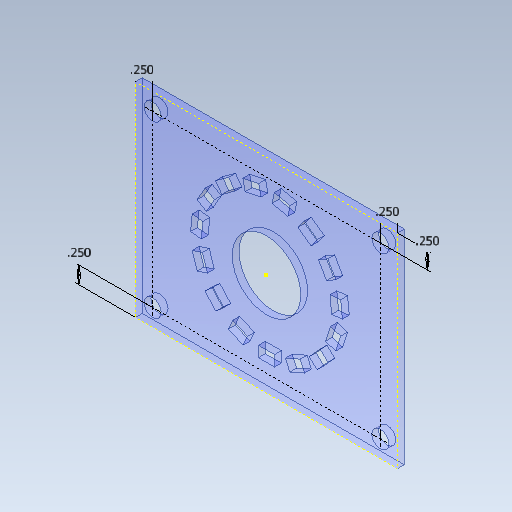
# Autodesk Inventor part: 2020LightRingCover
Saved by Autodesk Inventor 2020.2 (Build 242310000, 310)
## iProperties
Created: 2018-12-24
Part Number: 2020LightRingCover
Material: Polycarbonate, Clear
Document SubType Name: Modeling
Designer: steele
Density: 1.2 g/cm^3
Appearance: Clear - Blue
Author: steele
Comments: 1/11/19 Reduced the diamter of the outside by 2 mm so the part would fit better onto the main housing.
Autodesk Inventor part; units mm, degrees
ref_plane "YZ Plane" through (0, 0, 0) normal (1, 0, 0) x (0, 1, 0)
ref_plane "XZ Plane" through (0, 0, 0) normal (0, 1, 0) x (-1, 0, 0)
ref_plane "XY Plane" through (0, 0, 0) normal (0, 0, 1) x (1, 0, 0)
sketch "Sketch1" plane through (0, 0, 0) normal (0, 0, 1) x (1, 0, 0)
  circle A0 centre (0, 0) radius 34
  dimension "d0" = 68
  constraints: 1 centre point, 1 coincident
  measures "d0" diameter of A0
extrude "Extrusion1" add sketch "Sketch1" against normal blind 2.54
sketch "Sketch3" plane through (0, 0, -2.54) normal (0, 0, -1) x (-1, 0, 0)
  circle A0 centre (0, 0) radius 26 construction
  line L0 (3, -24) -> (-3, -24)
  line L1 (-3, -24) -> (-3, -28)
  line L2 (-3, -28) -> (3, -28)
  line L3 (3, -28) -> (3, -24)
  line L4 (3, -24) -> (-3, -28) construction
  line L5 (-3, -24) -> (3, -28) construction
  line L6 (8.648, -26.7995) -> (14.1293, -24.3591)
  line L7 (14.1293, -24.3591) -> (12.5023, -20.7049)
  line L8 (7.021, -23.1453) -> (8.648, -26.7995)
  line L9 (12.5023, -20.7049) -> (7.021, -23.1453)
  line L10 (18.8007, -20.9651) -> (22.8154, -16.5062)
  line L11 (22.8154, -16.5062) -> (19.8429, -13.8297)
  line L12 (15.8281, -18.2886) -> (18.8007, -20.9651)
  line L13 (19.8429, -13.8297) -> (15.8281, -18.2886)
  line L14 (25.7025, -11.5056) -> (27.5566, -5.7993)
  line L15 (27.5566, -5.7993) -> (23.7524, -4.5632)
  line L16 (21.8983, -10.2696) -> (25.7025, -11.5056)
  line L17 (23.7524, -4.5632) -> (21.8983, -10.2696)
  line L18 (28.1602, -0.0568) -> (27.533, 5.9104)
  line L19 (27.533, 5.9104) -> (23.5549, 5.4922)
  line L20 (24.1821, -0.4749) -> (28.1602, -0.0568)
  line L21 (23.5549, 5.4922) -> (24.1821, -0.4749)
  line L22 (25.7487, 11.4019) -> (22.7487, 16.5981)
  line L23 (22.7487, 16.5981) -> (19.2846, 14.5981)
  line L24 (22.2846, 9.4019) -> (25.7487, 11.4019)
  line L25 (19.2846, 14.5981) -> (22.2846, 9.4019)
  line L26 (18.885, 20.8891) -> (14.0309, 24.4158)
  line L27 (14.0309, 24.4158) -> (11.6798, 21.1798)
  line L28 (16.5339, 17.6531) -> (18.885, 20.8891)
  line L29 (11.6798, 21.1798) -> (16.5339, 17.6531)
  line L30 (8.756, 26.7644) -> (2.8871, 28.0119)
  line L31 (2.8871, 28.0119) -> (2.0554, 24.0993)
  line L32 (7.9243, 22.8518) -> (8.756, 26.7644)
  line L33 (2.0554, 24.0993) -> (7.9243, 22.8518)
  line L34 (-2.8871, 28.0119) -> (-8.756, 26.7644)
  line L35 (-8.756, 26.7644) -> (-7.9243, 22.8518)
  line L36 (-2.0554, 24.0993) -> (-2.8871, 28.0119)
  line L37 (-7.9243, 22.8518) -> (-2.0554, 24.0993)
  line L38 (-14.0309, 24.4158) -> (-18.885, 20.8891)
  line L39 (-18.885, 20.8891) -> (-16.5339, 17.6531)
  line L40 (-11.6798, 21.1798) -> (-14.0309, 24.4158)
  line L41 (-16.5339, 17.6531) -> (-11.6798, 21.1798)
  line L42 (-22.7487, 16.5981) -> (-25.7487, 11.4019)
  line L43 (-25.7487, 11.4019) -> (-22.2846, 9.4019)
  line L44 (-19.2846, 14.5981) -> (-22.7487, 16.5981)
  line L45 (-22.2846, 9.4019) -> (-19.2846, 14.5981)
  line L46 (-27.533, 5.9104) -> (-28.1602, -0.0568)
  line L47 (-28.1602, -0.0568) -> (-24.1821, -0.4749)
  line L48 (-23.5549, 5.4922) -> (-27.533, 5.9104)
  line L49 (-24.1821, -0.4749) -> (-23.5549, 5.4922)
  line L50 (-27.5566, -5.7993) -> (-25.7025, -11.5056)
  line L51 (-25.7025, -11.5056) -> (-21.8983, -10.2696)
  line L52 (-23.7524, -4.5632) -> (-27.5566, -5.7993)
  line L53 (-21.8983, -10.2696) -> (-23.7524, -4.5632)
  line L54 (-22.8154, -16.5062) -> (-18.8007, -20.9651)
  line L55 (-18.8007, -20.9651) -> (-15.8281, -18.2886)
  line L56 (-19.8429, -13.8297) -> (-22.8154, -16.5062)
  line L57 (-15.8281, -18.2886) -> (-19.8429, -13.8297)
  line L58 (-14.1293, -24.3591) -> (-8.648, -26.7995)
  line L59 (-8.648, -26.7995) -> (-7.021, -23.1453)
  line L60 (-12.5023, -20.7049) -> (-14.1293, -24.3591)
  line L61 (-7.021, -23.1453) -> (-12.5023, -20.7049)
  point P0 (0, -26)
  dimension "d6" = 52
  dimension "d7" = 4
  dimension "d8" = 6
  dimension "d11" = 360
  constraints: 124 end point, 2 midpoint, 2 parallel, 1 coincident, 1 horizontal, 1 perpendicular, 1 vertical alignment, 123 other
  measures "d7" distance of L2.end L0.start
  measures "d8" distance of L1.end L2.end
extrude "Extrusion3" cut sketch "Sketch3" against normal through all
sketch "Sketch7" plane through (0, 0, 0) normal (0, 0, 1) x (1, 0, 0)
  line L0 (-48.5775, -37.85) -> (48.5775, -37.85)
  line L1 (48.5775, -37.85) -> (48.5775, 37.85)
  line L2 (48.5775, 37.85) -> (-48.5775, 37.85)
  line L3 (-48.5775, 37.85) -> (-48.5775, -37.85)
  line L4 (-48.5775, -37.85) -> (48.5775, 37.85) construction
  line L5 (48.5775, -37.85) -> (-48.5775, 37.85) construction
  circle A0 centre (0, 0) radius 34
  dimension "mountWidth" = 97.155
  dimension "mountHeight" = 75.7
  constraints: 12 end point, 2 midpoint, 2 parallel, 1 centre point, 1 coincident, 1 horizontal, 1 perpendicular
  measures "mountWidth" distance of L0.start L0.end
  measures "mountHeight" distance of L2.end L0.start
extrude "Extrusion4" add sketch "Sketch7" against normal blind 2.54
sketch "Sketch8" plane through (0, 0, 0) normal (0, 0, 1) x (1, 0, 0)
  line L0 (-42.2275, -31.5) -> (42.2275, -31.5) construction
  line L1 (42.2275, -31.5) -> (42.2275, 31.5) construction
  line L2 (42.2275, 31.5) -> (-42.2275, 31.5) construction
  line L3 (-42.2275, 31.5) -> (-42.2275, -31.5) construction
  line L4 (-48.5775, -37.85) -> (48.5775, -37.85) construction
  line L5 (-48.5775, 37.85) -> (-48.5775, -37.85) construction
  line L6 (48.5775, -37.85) -> (48.5775, 37.85) construction
  line L7 (48.5775, 37.85) -> (-48.5775, 37.85) construction
  point P0 (0, 0)
  dimension "d47" = 6.35
  dimension "d48" = 6.35
  dimension "d49" = 6.35
  dimension "d50" = 6.35
  constraints: 8 end point, 4 coincident, 2 parallel, 1 horizontal, 1 perpendicular
  measures "d47" distance between parallel lines of L0 L4
  measures "d48" distance between parallel lines of L5 L3
  measures "d49" distance between parallel lines of L1 L6
  measures "d50" distance between parallel lines of L7 L2
sketch "Sketch10" plane through (0, 0, 0) normal (0, 0, 1) x (1, 0, 0)
  circle A0 centre (0, 0) radius 12.7
  dimension "d58" = 25.4
  constraints: 1 centre point, 1 coincident
  measures "d58" diameter of A0
extrude "Extrusion5" cut sketch "Sketch10" against normal through all
sketch "Sketch11" plane through (0, 0, 0) normal (0, 0, 1) x (1, 0, 0)
  circle A0 centre (-42.2275, 31.5) radius 2.5527 projected
  circle A1 centre (-42.2275, 31.5) radius 3.175
  circle A2 centre (42.2275, 31.5) radius 2.5527 projected
  circle A3 centre (42.2275, 31.5) radius 3.175
  circle A4 centre (42.2275, -31.5) radius 2.5527 projected
  circle A5 centre (42.2275, -31.5) radius 3.175
  circle A6 centre (-42.2275, -31.5) radius 2.5527 projected
  circle A7 centre (-42.2275, -31.5) radius 3.175
  point P0 (0, 0)
  dimension "d61" = 6.35
  constraints: 4 centre point, 4 coincident, 3 equal radius
  measures "d61" diameter of A1
extrude "Extrusion6" cut sketch "Sketch11" against normal through all contours A0 | A1 | A2 | A3 | A4 | A5 | A6 | A7
equation "\"d1\" = CoverDepth"
equation "\"d6\" = 2 * LightRingCenterRadius"
equation "\"depth\" = CoverDepth"
equation "\"CoverDepth\" = 2.54"
equation "\"LightRingCenterRadius\" = 26"
body "Solid1"
